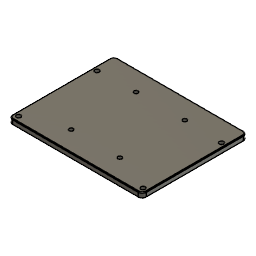
mid360_platform_v0_1 (Autodesk Fusion 360 design; units mm, degrees)
part number: 2026-06-01-13-28-28-103
Autodesk Fusion 360 part; units mm, degrees
box "长方体基本要素1" add length 77.8 width 98.8 height 4 placed x (0, 0, 1) y (1, 0, 0) z (0, 1, 0) at (0, 0, 0)
sketch "草图2" plane through (0, 4, 0) normal (0, 1, 0) x (-1, 0, 0)
  line L0 (0, 77.8) -> (-98.8, 77.8)
  line L1 (-98.8, 77.8) -> (-98.8, 0)
  line L2 (-98.8, 0) -> (0, 0)
  line L3 (0, 0) -> (0, 77.8)
  circle A0 centre (-3.4, 73.8) radius 1.6
  circle A1 centre (-3.4, 15.8) radius 1.6
  line L4 (-49.4, 0) -> (-49.4, 77.8) construction
  line L5 (-49.4, 0) -> (-49.4, 77.8) construction
  circle A2 centre (-95.4, 15.8) radius 1.6
  circle A3 centre (-95.4, 73.8) radius 1.6
  line L6 (-17.531, 7.031) -> (-81.269, 7.031)
  line L7 (-81.269, 7.031) -> (-81.269, 70.769)
  line L8 (-81.269, 70.769) -> (-17.531, 70.769)
  line L9 (-17.531, 70.769) -> (-17.531, 7.031)
  line L10 (0, 38.9) -> (-98.8, 38.9) construction
  circle A4 centre (-31.4, 62.9) radius 1.45
  circle A5 centre (-67.4, 62.9) radius 1.45
  circle A6 centre (-31.4, 14.9) radius 1.45
  circle A7 centre (-67.4, 14.9) radius 1.45
  circle A8 centre (-67.4, 62.9) radius 1.45
  circle A9 centre (-31.4, 14.9) radius 1.45
  circle A10 centre (-67.4, 14.9) radius 1.45
  line L11 (0, 77.8) -> (0.6, 77.8)
  line L12 (0.6, 77.8) -> (0.6, 0)
  line L13 (0.6, 0) -> (0, 0)
  line L14 (-99.4, 0) -> (-98.8, 0)
  line L15 (-99.4, 77.8) -> (-99.4, 0)
  line L16 (-98.8, 77.8) -> (-99.4, 77.8)
  dimension "d8" = 3.2
  dimension "d12" = 4
  dimension "d13" = 58
  dimension "d14" = 63.738
  dimension "d15" = 2.9
  dimension "d16" = 7.869
  dimension "d17" = 13.869
  dimension "d24" = 0.6
  dimension "d25" = 4
  constraint equal A0 A1
  constraint vertical A0.centre A1.centre
  constraint midpoint L2 L4.start
  constraint midpoint L0 L4.end
  constraint symmetric A0 L4 A3
  constraint symmetric A1 L4 A2
  constraint symmetric L5.start L4 L4.start
  constraint symmetric L5.end L4 L4.end
  constraint horizontal L6
  constraint vertical L7
  constraint horizontal L8
  constraint vertical L9
  constraint equal L6 L9
  constraint symmetric L5 L7 L9
  constraint midpoint L3 L10.start
  constraint midpoint L1 L10.end
  constraint symmetric L6 L8 L10
  constraint symmetric L5 A4 A5
  constraint symmetric L10 A4 A6
  constraint symmetric L10 A5 A7
  constraint symmetric L5 A4 A8
  constraint symmetric L10 A4 A9
  constraint symmetric L10 A8 A10
  constraint coincident L0.start L3.end
  constraint perpendicular L3 L11
  constraint perpendicular L2 L12
  constraint coincident L2.end L3.start
  constraint perpendicular L3 L13
  constraint symmetric L4 L0.start L0.end
  constraint symmetric L4 L11.end L15.start
  constraint symmetric L4 L12.end L14.start
  constraint symmetric L4 L2.end L1.end
  measures "d8" diameter of A0
  measures "d12" distance of L0 A0.centre
  measures "d13" distance of A0.centre A1.centre
  measures "d14" distance of L6.start L6.end
  measures "d15" diameter of A4
  measures "d16" distance of L8 A4.centre
  measures "d17" distance of L9 A4.centre
  measures "d24" distance of L0.start L11.end
  measures "d25" distance of A0.centre L12
fillet "圆角1" radius 3 4 edges at (98.8, 2, 77.8) (98.8, 2, 0) (0, 2, 0) (0, 2, 77.8)
fillet "圆角2" radius 0.5 16 edges at (0.8787, 4, 0.8787) (0, 4, 38.9) (0.8787, 4, 76.9213) (49.4, 4, 77.8) (97.9213, 4, 76.9213) (98.8, 4, 38.9) (97.9213, 4, 0.8787) (49.4, 4, 0) (97.9213, 0, 0.8787) (98.8, 0, 38.9) (97.9213, 0, 76.9213) (49.4, 0, 77.8) (0.8787, 0, 76.9213) (0, 0, 38.9) (0.8787, 0, 0.8787) (49.4, 0, 0)
extrude "拉伸1" cut sketch "草图2" against normal blind 4 contours A0 | A1 | A2 | A3 | A4 | A5 A8 | A6 A9 | A7 A10
